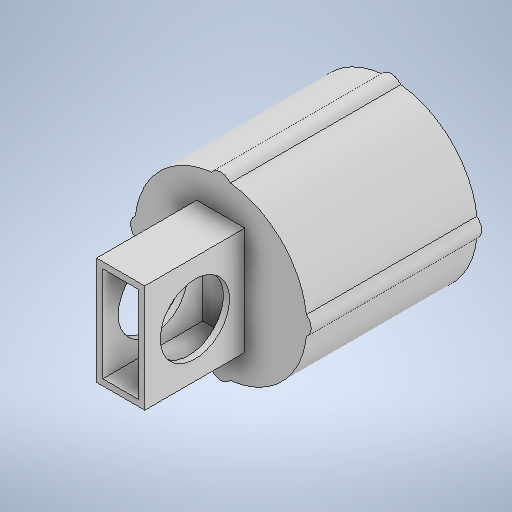
# Autodesk Inventor part: power_sensor_aperture_V1.1
Saved by Autodesk Inventor 2025.1 (Build 291241000, 241)
## iProperties
Created: 2023-11-21
Part Number: power_sensor_aperture_V1.1
Material: Generisch
Document SubType Name: Modeling
Designer: Daniel
Density: 1 g/cm^3
Appearance: Vorgabe
Author: Daniel
Autodesk Inventor part; units mm, degrees
ref_plane "YZ Plane" through (0, 0, 0) normal (1, 0, 0) x (0, 1, 0)
ref_plane "XZ Plane" through (0, 0, 0) normal (0, 1, 0) x (-1, 0, 0)
ref_plane "XY Plane" through (0, 0, 0) normal (0, 0, 1) x (1, 0, 0)
sketch "Sketch1" plane through (0, 0, 0) normal (0, 0, 1) x (1, 0, 0)
  circle A0 centre (0, 0) radius 11.25
  circle A1 centre (0, 0) radius 35.025
  circle A2 centre (0, 0) radius 37.030393
  arc A3 (-32.79294, -17.200962) -> (-31.29294, -19.799038) centre (0, 0) ccw
  line L0 (-32.79294, -17.200962) -> (-31.05471, -16.197395)
  line L1 (-32.79294, -17.200962) -> (-31.05471, -16.197395)
  line L2 (-29.55471, -18.795471) -> (-31.29294, -19.799038)
  line L3 (-31.29294, -19.799038) -> (-29.55471, -18.795471)
  line L4 (-16.197395, -31.05471) -> (-17.200962, -32.79294)
  line L5 (-17.200962, -32.79294) -> (-16.197395, -31.05471)
  arc A4 (-19.799038, -31.29294) -> (-17.200962, -32.79294) centre (0, 0) ccw
  line L6 (-19.799038, -31.29294) -> (-18.795471, -29.55471)
  line L7 (-19.799038, -31.29294) -> (-18.795471, -29.55471)
  arc A5 (17.200962, -32.79294) -> (19.799038, -31.29294) centre (0, 0) ccw
  line L8 (17.200962, -32.79294) -> (16.197395, -31.05471)
  line L9 (17.200962, -32.79294) -> (16.197395, -31.05471)
  line L10 (18.795471, -29.55471) -> (19.799038, -31.29294)
  line L11 (19.799038, -31.29294) -> (18.795471, -29.55471)
  arc A6 (31.29294, -19.799038) -> (32.79294, -17.200962) centre (0, 0) ccw
  line L12 (31.29294, -19.799038) -> (29.55471, -18.795471)
  line L13 (31.05471, -16.197395) -> (32.79294, -17.200962)
  line L14 (32.79294, -17.200962) -> (31.05471, -16.197395)
  line L15 (32.79294, 17.200962) -> (31.05471, 16.197395)
  line L16 (32.79294, 17.200962) -> (31.05471, 16.197395)
  arc A7 (32.79294, 17.200962) -> (31.29294, 19.799038) centre (0, 0) ccw
  line L17 (29.55471, 18.795471) -> (31.29294, 19.799038)
  line L18 (31.29294, 19.799038) -> (29.55471, 18.795471)
  line L19 (16.197395, 31.05471) -> (17.200962, 32.79294)
  line L20 (17.200962, 32.79294) -> (16.197395, 31.05471)
  line L21 (19.799038, 31.29294) -> (18.795471, 29.55471)
  line L22 (19.799038, 31.29294) -> (18.795471, 29.55471)
  line L23 (-17.200962, 32.79294) -> (-16.197395, 31.05471)
  line L24 (-17.200962, 32.79294) -> (-16.197395, 31.05471)
  line L25 (-18.795471, 29.55471) -> (-19.799038, 31.29294)
  line L26 (-19.799038, 31.29294) -> (-18.795471, 29.55471)
  arc A8 (-31.29294, 19.799038) -> (-32.79294, 17.200962) centre (0, 0) ccw
  line L27 (-31.29294, 19.799038) -> (-29.55471, 18.795471)
  line L28 (-31.29294, 19.799038) -> (-29.55471, 18.795471)
  line L29 (-31.05471, 16.197395) -> (-32.79294, 17.200962)
  line L30 (-32.79294, 17.200962) -> (-31.05471, 16.197395)
  arc A9 (-34.800207, -3.961848) -> (-34.800207, 3.961848) centre (-31.75, 0) ccw
  circle A10 centre (-31.75, 0) radius 5
  arc A11 (-3.961848, 34.800207) -> (3.961848, 34.800207) centre (0, 31.75) ccw
  circle A12 centre (0, 31.75) radius 5
  circle A13 centre (31.75, 0) radius 5
  circle A14 centre (31.75, 0) radius 5
  arc A15 (-3.961848, -34.800207) -> (3.961848, -34.800207) centre (0, -31.75) ccw
  circle A16 centre (0, -31.75) radius 5
  circle A17 centre (0, 31.75) radius 4.75
  circle A18 centre (-31.75, 0) radius 4.75
  circle A19 centre (0, -31.75) radius 4.75
  circle A20 centre (31.75, 0) radius 4.75
  circle A21 centre (0, 0) radius 34.775
  circle A22 centre (0, 0) radius 36.75
  point P0 (0, 0)
  point P1 (0, 49.75)
  point P2 (34.563789, -3.82689)
  point P3 (34.563789, 3.82689)
  point P4 (3.82689, 34.563789)
  point P5 (-3.82689, 34.563789)
  point P6 (-34.563789, 3.82689)
  point P7 (-34.563789, -3.82689)
  point P8 (-3.82689, -34.563789)
  point P9 (3.82689, -34.563789)
  dimension "d6" = 70.05
  dimension "d8" = 74.06079
  dimension "d0" = 10
  dimension "d1" = 0.25
  dimension "d4" = 360
  dimension "d7" = 0.25
  dimension "d9" = 73.5
  constraints: 62 end point, 21 centre point, 18 point on circle, 15 collinear, 10 coincident, 16 other
  measures "d0" diameter of A12
  measures "d1" radial gap between concentric circles of A12 A17
  measures "d9" diameter of A22
sketch "Sketch1 outline for Extrusion1" plane through (0, 0, 0) normal (0, 0, 1) x (1, 0, 0)
  arc A0 (3.82689, -34.563789) -> (34.563789, -3.82689) centre (0, 0) ccw
  arc A1 (-3.82689, -34.563789) -> (3.82689, -34.563789) centre (0, -31.75) ccw
  arc A2 (-34.563789, -3.82689) -> (-3.82689, -34.563789) centre (0, 0) ccw
  arc A3 (-34.563789, 3.82689) -> (-34.563789, -3.82689) centre (-31.75, 0) ccw
  arc A4 (-3.82689, 34.563789) -> (-34.563789, 3.82689) centre (0, 0) ccw
  arc A5 (3.82689, 34.563789) -> (-3.82689, 34.563789) centre (0, 31.75) ccw
  arc A6 (34.563789, 3.82689) -> (3.82689, 34.563789) centre (0, 0) ccw
  arc A7 (34.563789, -3.82689) -> (34.563789, 3.82689) centre (31.75, 0) ccw
extrude "Extrusion1" add sketch "Sketch1 outline for Extrusion1" along normal blind 68.9
sketch "Skizze4" plane through (0, 0, 68.9) normal (0, 0, 1) x (1, 0, 0)
  line L0 (-9.75, 21.75) -> (9.75, 21.75) construction
  line L1 (9.75, 21.75) -> (9.75, -21.75) construction
  line L2 (9.75, -21.75) -> (-9.75, -21.75) construction
  line L3 (-9.75, -21.75) -> (-9.75, 21.75) construction
  line L4 (-9.75, 21.75) -> (9.75, -21.75) construction
  line L5 (9.75, 21.75) -> (-9.75, -21.75) construction
  line L6 (-9.75, 21.75) -> (-7.25, 21.75)
  line L7 (-7.25, 21.75) -> (-7.25, -21.75)
  line L8 (-7.25, -21.75) -> (-9.75, -21.75)
  line L9 (-9.75, -21.75) -> (-9.75, 21.75)
  line L10 (9.75, 21.75) -> (7.25, 21.75)
  line L11 (7.25, 21.75) -> (7.25, -21.75)
  line L12 (7.25, -21.75) -> (9.75, -21.75)
  line L13 (9.75, -21.75) -> (9.75, 21.75)
  line L14 (-7.25, -21.75) -> (8.25, -21.75)
  line L15 (8.25, -21.75) -> (8.25, -19.25)
  line L16 (8.25, -19.25) -> (-7.25, -19.25)
  line L17 (-7.25, -19.25) -> (-7.25, -21.75)
  line L18 (-7.25, 21.75) -> (8.25, 21.75)
  line L19 (8.25, 21.75) -> (8.25, 19.25)
  line L20 (8.25, 19.25) -> (-7.25, 19.25)
  line L21 (-7.25, 19.25) -> (-7.25, 21.75)
  point P0 (0, 0)
  point P1 (7.25, 19.25)
  point P2 (7.25, -19.25)
  dimension "d24" = 19.5
  dimension "d25" = 43.5
  dimension "d26" = 2.5
  dimension "d27" = 2.5
  dimension "d28" = 15.5
  dimension "d29" = 2.5
  dimension "d30" = 15.5
  dimension "d31" = 2.5
  constraints: 44 end point, 10 parallel, 5 horizontal, 5 perpendicular, 2 midpoint, 2 point on line
  measures "d24" distance of L1.end L2.end
  measures "d25" distance of L0.end L1.end
  measures "d26" distance of L7.end L8.end
  measures "d27" distance of L12.end L11.end
  measures "d28" distance of L16.end L15.end
  measures "d29" distance of L15.end L14.end
  measures "d30" distance of L19.end L20.end
  measures "d31" distance of L18.end L19.end
extrude "Extrusion4" add sketch "Skizze4" along normal blind 40.5 contours L6 L7 L8 L9 | L18 L11 L20 L7 | L10 L19 L20 L11 | L7 L16 L11 L14 | L20 L19 L10 L13 L12 L15 L16 L11 | L11 L16 L15 L12
sketch "Skizze5" plane through (9.75, -21.75, 68.9) normal (1, 0, 0) x (0, 0, -1)
  line L0 (-40.5, 43.5) -> (-40.5, 0) construction
  line L1 (0, 0) -> (-40.5, 0) construction
  line L2 (-40.5, 43.5) -> (0, 0) construction
  line L3 (0, 43.5) -> (-40.5, 43.5) construction
  line L4 (0, 43.5) -> (-40.5, 0) construction
  circle A0 centre (-20.25, 21.75) radius 14
  point P0 (68.9, 21.75)
  dimension "d35" = 28
  constraints: 4 end point, 2 midpoint, 1 centre point
  measures "d35" diameter of A0
extrude "Extrusion5" cut sketch "Skizze5" against normal through all
body "Solid1"
